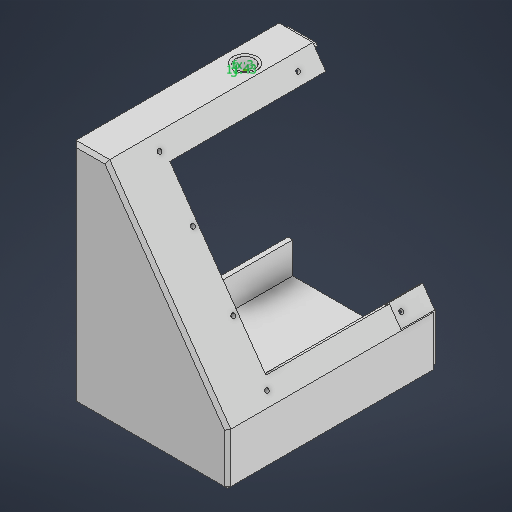
# Autodesk Inventor part: case3
Saved by Autodesk Inventor 2026.2 (Build 302298000, 298)
## iProperties
Created: 2026-01-28
Part Number: case3
Material: Generic
Document SubType Name: Modeling
Designer: test
Density: 1 g/cm^3
Appearance: Default
Author: test
## iProperties of the stored document case3_3DPrint.ipt
Created: 2026-01-28
Part Number: case3_3DPrint
Material: Generic
Document SubType Name: Modeling
Designer: test
Density: 1 g/cm^3
Appearance: Default
Author: test
Autodesk Inventor part; units mm, degrees
ref_plane "YZ Plane" through (0, 0, 0) normal (1, 0, 0) x (0, 1, 0)
ref_plane "XZ Plane" through (0, 0, 0) normal (0, 1, 0) x (-1, 0, 0)
ref_plane "XY Plane" through (0, 0, 0) normal (0, 0, 1) x (1, 0, 0)
sketch "Sketch1" plane through (0, 0, 0) normal (0, 0, 1) x (1, 0, 0)
  line L0 (0, 0) -> (0, 199.7346)
  line L1 (0, 199.7346) -> (20, 199.7346)
  line L2 (20, 199.7346) -> (131.8474, 40)
  line L3 (131.8474, 40) -> (131.8474, 0)
  line L4 (131.8474, 0) -> (0, 0)
  dimension "d0" = 40
  dimension "d1" = 55
  dimension "d2" = 20
  dimension "d3" = 195
  constraints: 10 end point, 2 perpendicular, 1 parallel, 1 vertical
  measures "d0" distance of L2.end L3.end
  measures "d1" angle of L4 L2
  measures "d2" distance of L0.end L1.end
  measures "d3" distance of L1.end L2.end
extrude "Extrusion1" add sketch "Sketch1" against normal blind 189
sketch "Sketch5" plane through (131.8474, 40, 0) normal (0.819152, 0.5735764, 0) x (0, 0, -1)
  line L0 (189, 42.8585) -> (189, 206.4715) projected
  line L1 (189, 177.5) -> (40, 177.5)
  line L2 (40, 177.5) -> (40, 17.5)
  line L3 (40, 17.5) -> (189, 17.5)
  line L4 (189, 17.5) -> (189, 177.5)
  line L5 (0, 0) -> (0, 195) projected
  line L6 (0, 195) -> (189, 195) projected
  line L7 (0, 0) -> (189, 0) projected
  line L8 (0, 97.5) -> (189, 97.5) construction
  point P0 (0, 42.8585)
  point P1 (189, 42.8585)
  point P2 (40, 97.5)
  dimension "d30" = 40
  dimension "d33" = 160
  constraints: 10 end point, 3 midpoint, 2 parallel, 2 point on line, 1 horizontal, 1 perpendicular
  measures "d30" distance between parallel lines of L5 L2
  measures "d33" distance between parallel lines of L3 L1
extrude "Extrusion5" cut sketch "Sketch5" against normal blind 10
shell "Shell2" thickness 8 outward yes removed faces 5 at (45.1537, 76.0869, -189) at (52.4352, 135.9745, -89.6667) at (119.0788, 52.4229, -89.6667) at (27.3065, 183.4872, -139.3333) at (57.8973, 139.7991, -40)
sketch "Sketch3" plane through (25.2057, 209.7346, 10) normal (0.819152, 0.5735764, 0) x (0, 0, -1)
  line L0 (199, -1.0411) -> (199, -22.7057) projected
  line L1 (2, -1.0411) -> (199, -1.0411) projected
  line L2 (2, -202.7281) -> (2, -1.0411) projected
  line L3 (2, -202.7281) -> (199, -202.7281) projected
  line L4 (199, -182.7057) -> (199, -202.7281) projected
  line L5 (50, -102.7057) -> (132.4081, -102.7057) construction
  circle A0 centre (45.5, -69.2057) radius 2
  circle A1 centre (45.5, -13.2057) radius 2
  circle A2 centre (45.5, -136.2057) radius 2
  circle A3 centre (45.5, -192.2057) radius 2
  line L6 (45.5, -78.6989) -> (45.5, -69.2057) construction
  line L7 (199, -182.7057) -> (50, -182.7057) projected
  line L8 (50, -182.7057) -> (50, -22.7057) projected
  line L9 (50, -22.7057) -> (199, -22.7057) projected
  line L10 (50, -182.7057) -> (50, -22.7057) projected
  line L11 (50, -22.7057) -> (199, -22.7057) projected
  line L12 (199, -182.7057) -> (50, -182.7057) projected
  line L13 (45.5, -192.2057) -> (45.5, -13.2057) construction
  line L14 (10, -200.2057) -> (199, -200.2057) projected
  point P0 (10, -157.3472)
  point P1 (199, -12.2077)
  dimension "d22" = 4
  dimension "d23" = 4
  dimension "d24" = 4
  dimension "d25" = 4
  dimension "d35" = 179
  dimension "d43" = 67
  dimension "d45" = 4.5
  constraints: 6 end point, 4 centre point, 3 point on line, 2 symmetric about line, 1 coincident, 1 midpoint, 1 perpendicular
  measures "d22" diameter of A3
  measures "d23" diameter of A2
  measures "d24" diameter of A0
  measures "d25" diameter of A1
  measures "d35" distance of A3.centre L13.end
  measures "d43" distance of A2.centre L6.end
  measures "d45" distance between parallel lines of L13 L8
extrude "Extrusion4" cut sketch "Sketch3" against normal up to surface (10 mm away) contours A0 | A1 | A2 | A3
sketch "Sketch6" plane through (0, 0, -189) normal (0, 0, -1) x (-1, 0, 0)
  line L0 (-30.0376, 185.3995) -> (-20, 199.7346) projected
  line L1 (-20, 199.7346) -> (0, 199.7346) projected
  line L2 (0, 199.7346) -> (0, 0) projected
  line L3 (0, 0) -> (-131.8474, 0) projected
  line L4 (-131.8474, 0) -> (-131.8474, 40) projected
  line L5 (-131.8474, 40) -> (-121.8098, 54.3352) projected
  line L6 (-121.8098, 54.3352) -> (-128.363, 58.9238) projected
  line L7 (-128.363, 58.9238) -> (-139.8474, 42.5224) projected
  line L8 (-139.8474, 42.5224) -> (-139.8474, -8) projected
  line L9 (-139.8474, -8) -> (8, -8) projected
  line L10 (8, -8) -> (8, 207.7346) projected
  line L11 (8, 207.7346) -> (-24.1645, 207.7346) projected
  line L12 (-24.1645, 207.7346) -> (-36.5908, 189.9881) projected
  line L13 (-36.5908, 189.9881) -> (-30.0376, 185.3995) projected
  line L14 (4.5, 204.2346) -> (-22.3426, 204.2346)
  line L15 (-22.3426, 204.2346) -> (-33.7238, 187.9806)
  line L16 (-125.496, 56.9163) -> (-136.3474, 41.4188)
  line L17 (-136.3474, 41.4188) -> (-136.3474, -4.5)
  line L18 (-136.3474, -4.5) -> (4.5, -4.5)
  line L19 (4.5, -4.5) -> (4.5, 204.2346)
  dimension "d38" = 4.5
  dimension "d39" = 4.5
  constraints: 12 end point, 2 point on line, 4 other
  measures "d38" distance between parallel lines of L14 L1
  measures "d39" distance between parallel lines of L2 L19
extrude "Extrusion6" add sketch "Sketch6" along normal blind 5 contours L13 L15 L14 L19 L18 L17 L16 L6 L5 L4 L3 L2 L1 L0
sketch "Sketch7" plane through (24.1645, 207.7346, 8) normal (0.819152, 0.5735764, 0) x (0, 0, -1)
  circle A0 centre (43.5, -68.1645) radius 2 projected
  circle A1 centre (43.5, -135.1645) radius 2 projected
  circle A2 centre (43.5, -12.1645) radius 2 projected
  circle A3 centre (43.5, -191.1645) radius 2 projected
  line L0 (197, -181.6645) -> (48, -181.6645) projected
  line L1 (48, -181.6645) -> (48, -21.6645) projected
  line L2 (48, -21.6645) -> (197, -21.6645) projected
  line L3 (197, 0) -> (197, -21.6645) projected
  line L4 (0, 0) -> (197, 0) projected
  line L5 (0, -201.6869) -> (0, 0) projected
  line L6 (0, -201.6869) -> (197, -201.6869) projected
  line L7 (197, -181.6645) -> (197, -201.6869) projected
  line L8 (43.5, -12.1645) -> (176.055, -12.1645) construction
  line L9 (176.055, -12.1645) -> (176.055, -191.1645) construction
  line L10 (176.055, -191.1645) -> (43.5, -191.1645) construction
  line L11 (43.5, -191.1645) -> (43.5, -12.1645) construction
  circle A4 centre (176.055, -12.1645) radius 2
  circle A5 centre (176.055, -191.1645) radius 2
  point P0 (8, -156.3061)
  dimension "d46" = 132.555
  dimension "d47" = 4
  dimension "d48" = 4
  constraints: 8 end point, 3 coincident, 2 centre point, 2 parallel, 1 horizontal, 1 perpendicular
  measures "d46" distance of L9.end L10.end
  measures "d47" diameter of A4
  measures "d48" diameter of A5
extrude "Extrusion7" cut sketch "Sketch7" against normal up to surface (8 mm away) contours A4 | A5
sketch "Sketch8" plane through (131.8474, 40, -194) normal (-0.819152, -0.5735764, 0) x (0, 0, 1)
  circle A0 centre (25.945, 8) radius 2 projected
  circle A1 centre (25.945, 187) radius 2 projected
  circle A2 centre (158.5, 131) radius 2 projected
  circle A3 centre (158.5, 64) radius 2 projected
  circle A4 centre (158.5, 187) radius 2 projected
  circle A5 centre (158.5, 8) radius 2 projected
  line L0 (0, 17.5) -> (154, 17.5) projected
  line L1 (0, 0) -> (0, 17.5) projected
  line L2 (194, 0) -> (0, 0) projected
  line L3 (194, 0) -> (194, 195) projected
  line L4 (194, 195) -> (0, 195) projected
  line L5 (0, 177.5) -> (0, 195) projected
  line L6 (154, 177.5) -> (0, 177.5) projected
  line L7 (154, 17.5) -> (154, 177.5) projected
  line L8 (0, 177.5) -> (35.945, 177.5)
  line L9 (35.945, 177.5) -> (35.945, 195)
  line L10 (35.945, 195) -> (0, 195)
  line L11 (0, 195) -> (0, 177.5)
  point P0 (194, 42.8585)
  dimension "d51" = 10
  constraints: 8 end point, 2 parallel, 1 horizontal, 1 perpendicular, 1 point on line
  measures "d51" distance from line of A1.centre L9
extrude "Extrusion8" cut sketch "Sketch8" against normal blind 5 contours L6 L5 L4 L9
sketch "Sketch9" plane through (24.1645, 207.7346, 8) normal (0.819152, 0.5735764, 0) x (0, 0, -1)
  circle A0 centre (176.055, -191.1645) radius 2 projected
  circle A1 centre (176.055, -12.1645) radius 2 projected
  circle A2 centre (43.5, -68.1645) radius 2 projected
  circle A3 centre (43.5, -135.1645) radius 2 projected
  circle A4 centre (43.5, -12.1645) radius 2 projected
  circle A5 centre (43.5, -191.1645) radius 2 projected
  line L0 (197, -181.6645) -> (48, -181.6645) projected
  line L1 (48, -181.6645) -> (48, -21.6645) projected
  line L2 (48, -21.6645) -> (197, -21.6645) projected
  line L3 (197, 0) -> (197, -21.6645) projected
  line L4 (0, 0) -> (197, 0) projected
  line L5 (0, -201.6869) -> (0, 0) projected
  line L6 (0, -201.6869) -> (197, -201.6869) projected
  line L7 (197, -181.6645) -> (197, -201.6869) projected
  line L8 (197, -201.6869) -> (166.055, -201.6869)
  line L9 (166.055, -201.6869) -> (166.055, -181.6645)
  line L10 (166.055, -181.6645) -> (197, -181.6645)
  line L11 (197, -181.6645) -> (197, -201.6869)
  line L12 (197, -181.6645) -> (202, -181.6645) projected
  line L13 (197, -181.6645) -> (202, -181.6645)
  line L14 (202, -181.6645) -> (202, -201.6869)
  line L15 (202, -201.6869) -> (197, -201.6869)
  line L16 (197, -201.6869) -> (197, -181.6645)
  line L17 (202, -181.6645) -> (202, -200.5834) projected
  point P0 (8, -156.3061)
  dimension "d54" = 10
  constraints: 16 end point, 4 parallel, 3 point on line, 2 horizontal, 2 perpendicular
  measures "d54" distance from line of A0.centre L9
extrude "Extrusion9" cut sketch "Sketch9" against normal blind 5 contours L7 L6 L9 L0 | L12 L14 L15 L7
sketch "Sketch10" plane through (-8, -8, 8) normal (-1, 0, 0) x (0, 0, 1)
  line L0 (-61.055, 182.8673) -> (-271.055, 182.8673)
  line L1 (-291.055, 162.8673) -> (-291.055, 52.8673)
  line L2 (-271.055, 32.8673) -> (-61.055, 32.8673)
  line L3 (-41.055, 52.8673) -> (-41.055, 162.8673)
  line L4 (0, 215.7346) -> (0, 0) projected
  line L5 (0, 107.8673) -> (-197, 107.8673) construction
  line L6 (-197, 212.2346) -> (-197, 3.5) projected
  arc A0 (-61.055, 32.8673) -> (-41.055, 52.8673) centre (-61.055, 52.8673) ccw
  arc A1 (-41.055, 162.8673) -> (-61.055, 182.8673) centre (-61.055, 162.8673) ccw
  arc A2 (-271.055, 182.8673) -> (-291.055, 162.8673) centre (-271.055, 162.8673) ccw
  arc A3 (-291.055, 52.8673) -> (-271.055, 32.8673) centre (-271.055, 52.8673) ccw
  point P0 (-8, 8)
  point P1 (-166.055, 32.8673)
  point P2 (-41.055, 107.8673)
  dimension "d57" = 250
  dimension "d58" = 150
  dimension "d59" = 166.055
  dimension "d60" = 20
  constraints: 10 end point, 8 point on circle, 8 tangent, 4 centre point, 4 midpoint, 3 equal radius, 2 parallel, 2 perpendicular, 1 horizontal, 1 point on line
  measures "d57" distance between parallel lines of L3 L1
  measures "d58" distance between parallel lines of L0 L2
  measures "d59" distance from line of point (-166.055, 32.867) L4
  measures "d60" radius of A0
extrude "Extrusion10" cut sketch "Sketch10" against normal blind 3.5
sketch "Sketch11" plane through (-4.5, -4.5, -194) normal (-1, 0, 0) x (0, 0, 1)
  line L0 (0, 0) -> (0, 208.7346) projected
  line L1 (5, 0) -> (0, 0) projected
  line L2 (5, 29.3673) -> (5, 0) projected
  line L3 (140.945, 29.3673) -> (5, 29.3673) projected
  arc A0 (140.945, 29.3673) -> (160.945, 49.3673) centre (140.945, 49.3673) ccw projected
  line L4 (160.945, 159.3673) -> (160.945, 49.3673) projected
  arc A1 (160.945, 159.3673) -> (140.945, 179.3673) centre (140.945, 159.3673) ccw projected
  line L5 (5, 179.3673) -> (140.945, 179.3673) projected
  line L6 (5, 208.7346) -> (5, 179.3673) projected
  line L7 (5, 208.7346) -> (0, 208.7346) projected
  line L8 (5, 179.3673) -> (0, 179.3673)
  line L9 (0, 179.3673) -> (0, 29.3673)
  line L10 (0, 29.3673) -> (5, 29.3673)
  line L11 (5, 29.3673) -> (5, 179.3673)
  arc A2 (155.945, 159.3673) -> (140.945, 174.3673) centre (140.945, 159.3673) ccw
  line L12 (155.945, 159.3673) -> (155.945, 49.3673)
  arc A3 (140.945, 34.3673) -> (155.945, 49.3673) centre (140.945, 49.3673) ccw
  line L13 (140.945, 34.3673) -> (5, 34.3673)
  line L14 (5, 34.3673) -> (5, 174.3673)
  line L15 (5, 174.3673) -> (140.945, 174.3673)
  line L16 (5, 174.3673) -> (0, 174.3673)
  line L17 (0, 174.3673) -> (0, 34.3673)
  line L18 (0, 34.3673) -> (5, 34.3673)
  line L19 (5, 34.3673) -> (5, 174.3673)
  line L20 (155.945, 94.3673) -> (140.945, 94.3673)
  line L21 (140.945, 94.3673) -> (140.945, 114.3673)
  line L22 (140.945, 114.3673) -> (155.945, 114.3673)
  line L23 (155.945, 114.3673) -> (155.945, 94.3673)
  circle A4 centre (148.445, 104.3673) radius 2.5
  line L24 (140.945, 114.3673) -> (148.445, 114.3673) construction
  line L25 (148.445, 114.3673) -> (148.445, 104.3673) construction
  line L26 (148.445, 104.3673) -> (140.945, 104.3673) construction
  line L27 (140.945, 104.3673) -> (140.945, 114.3673) construction
  point P0 (194, 4.5)
  point P1 (0, 34.3673)
  point P2 (155.945, 104.3673)
  dimension "d63" = 5
  dimension "d70" = 20
  dimension "d71" = 20
  dimension "d72" = 10
  dimension "d73" = 7.5
  dimension "d74" = 5
  constraints: 40 end point, 8 parallel, 4 horizontal, 4 perpendicular, 4 point on circle, 3 centre point, 3 point on line, 2 midpoint, 5 other
  measures "d63" distance between parallel lines of L5 L15
  measures "d70" distance of L21.end L20.end
  measures "d71" distance between parallel lines of L4 L21
  measures "d72" distance between parallel lines of L26 L22
  measures "d73" distance between parallel lines of L25 L27
  measures "d74" diameter of A4
extrude "Extrusion11" cut sketch "Sketch11" against normal up to surface (4.5 mm away) contours L0 L16 L11 L18 | L11 L15 A2 L12 L22 L21 L20 A3 L13 | A4
fillet "Fillet3" radius 5 4 edges at (-2.25, 109.8673, -53.055) (-2.25, 89.8673, -53.055) (-2.25, 89.8673, -38.055) (-2.25, 109.8673, -38.055)
chamfer "Chamfer1" distance 3 angle 45 7 edges at (-8, 99.8673, 8) (8.0823, 207.7346, 8) (82.006, 125.1285, 8) (65.9237, -8, 8) (-8, -8, -90.5) (139.8474, -8, -90.5) (139.8474, 17.2612, 8)
sketch "Sketch13" plane through (0, 199.7346, 0) normal (0, -1, 0) x (1, 0, 0)
  line L0 (20, 0) -> (0, 0) projected
  line L1 (0, 0) -> (0, -194) projected
  line L2 (20, -194) -> (0, -194) projected
  line L3 (20, -158.055) -> (20, -194) projected
  line L4 (20, 0) -> (20, -158.055) projected
  line L5 (15.5919, -130.8427) -> (2.5919, -130.8427)
  line L6 (2.5919, -130.8427) -> (2.5919, -147.8427)
  line L7 (2.5919, -147.8427) -> (15.5919, -147.8427)
  line L8 (15.5919, -147.8427) -> (15.5919, -130.8427)
  circle A0 centre (9.0919, -139.3427) radius 1
  line L9 (15.5919, -130.8427) -> (9.0919, -130.8427) construction
  line L10 (9.0919, -130.8427) -> (9.0919, -139.3427) construction
  line L11 (9.0919, -139.3427) -> (15.5919, -139.3427) construction
  line L12 (15.5919, -139.3427) -> (15.5919, -130.8427) construction
  circle A1 centre (13.1809, -133.4919) radius 0.636
  circle A2 centre (13.5686, -144.6603) radius 0.8584
  point P0 (0, 0)
  dimension "d79" = 17
  dimension "d80" = 13
  dimension "d81" = 8.5
  dimension "d82" = 6.5
  dimension "d83" = 2
  constraints: 16 end point, 4 parallel, 3 centre point, 2 horizontal, 2 perpendicular
  measures "d79" distance between parallel lines of L7 L5
  measures "d80" distance between parallel lines of L6 L8
  measures "d81" distance between parallel lines of L5 L11
  measures "d82" distance between parallel lines of L8 L10
  measures "d83" diameter of A0
extrude "Extrusion12" cut sketch "Sketch13" against normal blind 2 contours L8 L7 L6 L5 | A0 | A1 | A2
extrude "Extrusion13" cut sketch "Sketch13" against normal up to surface (8 mm away) contours A0
ref_plane "Work Plane1" through (9.0919, 199.7346, -139.3427) normal (0, 0, -1) x (0, 1, 0)
sketch "Sketch14" plane through (9.0919, 199.7346, -139.3427) normal (0, 0, -1) x (0, 1, 0)
  line L0 (2, -1) -> (2, 1) projected
  line L1 (8, 1) -> (8, -1) projected
  line L2 (8, 15.0726) -> (8, -17.0919) projected
  line L3 (2, -1) -> (8, -1) projected
  line L4 (3, -1) -> (8, -10)
  line L5 (-250.8816, 0) -> (51.1469, 0) projected
  point P0 (-199.7346, -9.0919)
  dimension "d86" = 1
  dimension "d88" = 9
  constraints: 2 end point, 2 point on line
  measures "d86" distance from line of L0 L4.start
  measures "d88" distance from line of L3 L4.end
revolve "Revolution1" cut sketch "Sketch14" angle 360 about axis through (9.0919, 199.7346, -139.3427) along (0, 1, 0) contours L3 L2 L4
fillet "Fillet2" radius 5 1 edges at (19.0919, 207.7346, -139.3427)
sketch "Sketch15" plane through (0, 201.7346, 0) normal (0, -1, 0) x (1, 0, 0)
  circle A0 centre (9.0919, -139.3427) radius 1 projected
  line L0 (2.5919, -147.8427) -> (2.5919, -130.8427) projected
  line L1 (15.5919, -147.8427) -> (2.5919, -147.8427) projected
  line L2 (15.5919, -130.8427) -> (15.5919, -147.8427) projected
  line L3 (2.5919, -130.8427) -> (15.5919, -130.8427) projected
  circle A1 centre (5.577, -144.9573) radius 1.5
  circle A2 centre (5.577, -133.5273) radius 1.5
  line L4 (5.577, -144.9573) -> (5.577, -133.5273)
  line L5 (12.7098, -146.2282) -> (14.1639, -146.2282)
  line L6 (14.1639, -146.2282) -> (14.1639, -132.6966)
  line L7 (14.1639, -132.6966) -> (12.7098, -132.6966)
  line L8 (12.7098, -132.6966) -> (12.7098, -146.2282)
  point P0 (0, 0)
  dimension "d91" = 11.43
  dimension "d92" = 3
  dimension "d93" = 3
  constraints: 10 end point, 3 parallel, 2 centre point, 1 horizontal, 1 perpendicular, 1 vertical
  measures "d91" distance of L4.end L4.start
  measures "d92" diameter of A2
  measures "d93" diameter of A1
sketch "Sketch16" plane through (0, 0, 0) normal (0, 1, 0) x (1, 0, 0)
  line L0 (0, 0) -> (131.8474, 0) projected
  line L1 (131.8474, 0) -> (131.8474, 194) projected
  line L2 (0, 194) -> (131.8474, 194) projected
  line L3 (0, 0) -> (0, 194) projected
  line L4 (69, 128.5) -> (11, 128.5) construction
  line L5 (11, 128.5) -> (11, 79.5) construction
  line L6 (11, 79.5) -> (69, 79.5) construction
  line L7 (69, 79.5) -> (69, 128.5) construction
  circle A0 centre (69, 128.5) radius 1.25
  circle A1 centre (69, 79.5) radius 1.25
  circle A2 centre (11, 79.5) radius 1.25
  circle A3 centre (11, 128.5) radius 1.25
  line L8 (131.8474, 194) -> (40, 194) construction
  line L9 (40, 194) -> (40, 104) construction
  line L10 (40, 104) -> (131.8474, 104) construction
  line L11 (131.8474, 104) -> (131.8474, 194) construction
  point P0 (40, 128.5)
  point P1 (69, 104)
  dimension "d94" = 58
  dimension "d95" = 49
  dimension "d96" = 2.5
  dimension "d97" = 2.5
  dimension "d98" = 2.5
  dimension "d99" = 2.5
  dimension "d100" = 40
  dimension "d101" = 90
  constraints: 16 end point, 4 centre point, 4 coincident, 4 parallel, 2 horizontal, 2 midpoint, 2 perpendicular, 2 point on line
  measures "d94" distance between parallel lines of L5 L7
  measures "d95" distance between parallel lines of L4 L6
  measures "d96" diameter of A0
  measures "d97" diameter of A1
  measures "d98" diameter of A2
  measures "d99" diameter of A3
  measures "d100" distance between parallel lines of L3 L9
  measures "d101" distance between parallel lines of L2 L10
extrude "Extrusion14" cut sketch "Sketch16" against normal blind 5 contours A0 | A1 | A2 | A3
equation "\"d23\" = d22"
equation "\"d39\" = d38"
body "Solid1"
